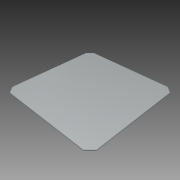
# Autodesk Inventor part: heatbed_glass_top
Saved by Autodesk Inventor 2014 (Build 180170000, 170)
## iProperties
Created: 2013-11-29
Part Number: heatbed_glass_top
Material: Glass
Document SubType Name: Modeling
Designer: buben
Density: 2.18 g/cm^3
Appearance: Clear
Author: buben
Autodesk Inventor part; units mm, degrees
ref_plane "YZ Plane" through (0, 0, 0) normal (1, 0, 0) x (0, 1, 0)
ref_plane "XZ Plane" through (0, 0, 0) normal (0, 1, 0) x (-1, 0, 0)
ref_plane "XY Plane" through (0, 0, 0) normal (0, 0, 1) x (1, 0, 0)
sketch "Sketch1" plane through (0, 0, 0) normal (0, 0, 1) x (1, 0, 0)
  line L0 (13, 0) -> (203, 0)
  line L1 (216, 13) -> (216, 203)
  line L2 (203, 216) -> (13, 216)
  line L3 (0, 203) -> (0, 13)
  line L4 (0, 13) -> (13, 0)
  line L5 (203, 0) -> (216, 13)
  line L6 (216, 203) -> (203, 216)
  line L7 (13, 216) -> (0, 203)
  point P0 (0, 0)
  point P1 (216, 216)
  point P2 (216, 0)
  point P3 (0, 216)
  dimension "d0" = 216
  dimension "d1" = 216
  dimension "d2" = 13
  dimension "d3" = 13
  dimension "d4" = 13
  dimension "d5" = 13
  dimension "d6" = 13
  dimension "d7" = 13
  dimension "d8" = 13
  dimension "d9" = 13
  constraints: 16 end point, 8 point on line, 2 parallel, 1 horizontal, 1 perpendicular
  measures "d0" distance of point (0, 216) point (0, 0)
  measures "d1" distance of point (0, 0) point (216, 0)
  measures "d2" distance of L3.end point (0, 0)
  measures "d3" distance of L0.start point (0, 0)
  measures "d4" distance of L0.end point (216, 0)
  measures "d5" distance of L1.start point (216, 0)
  measures "d6" distance of L1.end point (216, 216)
  measures "d7" distance of L2.start point (216, 216)
  measures "d8" distance of L2.end point (0, 216)
  measures "d9" distance of L3.start point (0, 216)
extrude "Extrusion1" add sketch "Sketch1" along normal blind 2
chamfer "Chamfer1" distance 0.5 angle 45 24 edges at (108, 0, 2) (6.5, 6.5, 2) (0, 108, 2) (6.5, 209.5, 2) (108, 216, 2) (209.5, 209.5, 2) (216, 108, 2) (209.5, 6.5, 2) (209.5, 6.5, 0) (216, 108, 0) (108, 0, 0) (6.5, 6.5, 0) (0, 108, 0) (6.5, 209.5, 0) (108, 216, 0) (209.5, 209.5, 0) (216, 203, 1) (203, 216, 1) (13, 216, 1) (0, 203, 1) (13, 0, 1) (0, 13, 1) (216, 13, 1) (203, 0, 1)
equation "\"d3\" = d2"
equation "\"d4\" = d2"
equation "\"d5\" = d4"
equation "\"d6\" = d2"
equation "\"d7\" = d6"
equation "\"d8\" = d2"
equation "\"d9\" = d8"
body "Solid1"
